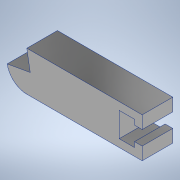
# Autodesk Inventor part: Finray_test_8
Saved by Autodesk Inventor 2022 (Build 260153000, 153)
## iProperties
Created: 2022-02-28
Part Number: Finray_test_8
Material: Generic
Document SubType Name: Modeling
Designer: richa
Density: 1 g/cm^3
Appearance: Aluminum - Flat
Author: richa
Autodesk Inventor part; units mm, degrees
ref_plane "YZ Plane" through (0, 0, 0) normal (1, 0, 0) x (0, 1, 0)
ref_plane "XZ Plane" through (0, 0, 0) normal (0, 1, 0) x (-1, 0, 0)
ref_plane "XY Plane" through (0, 0, 0) normal (0, 0, 1) x (1, 0, 0)
sketch "Sketch5" plane through (0, 0, 0) normal (0, 0, 1) x (1, 0, 0)
  line L0 (53, -15.6) -> (53, -10.6)
  line L1 (53, -10.6) -> (50, -10.6)
  line L2 (50, -10.6) -> (50, -12.6)
  line L3 (44, -12.6) -> (44, -3)
  line L4 (50, -3) -> (50, -5)
  line L5 (50, -5) -> (53, -5)
  line L6 (53, -5) -> (53, 0)
  line L7 (53, 0) -> (7.8, 0)
  line L8 (44, -3) -> (50, -3)
  line L9 (44, -12.6) -> (50, -12.6)
  line L10 (53, -15.6) -> (7.8, -15.6)
  arc A0 (7.8, 0) -> (7.8, -15.6) centre (7.8, -7.8) ccw
  point P0 (0, 0)
  dimension "d41" = 6
  dimension "d48" = 44
  dimension "d50" = 3
  dimension "d63" = 45.2
  dimension "d67" = 15.6
  dimension "d71" = 0
  dimension "d72" = 36.2
  dimension "d73" = 5
  dimension "d75" = 5
  dimension "d76" = 3
  dimension "d77" = 3
  constraints: 22 end point, 7 perpendicular, 2 collinear, 2 parallel, 2 point on circle, 2 tangent, 1 centre point, 1 horizontal, 1 vertical
  measures "d41" distance between parallel lines of L2 L3
  measures "d48" distance from line of L3 point (0, 0)
  measures "d50" distance of L4.end L5.end
  measures "d63" distance of L0.start L10.end
  measures "d67" diameter of A0
  measures "d71" distance from line of point (0, 0) L7
  measures "d72" distance from line of L3 A0.centre
  measures "d73" distance of L0.start L0.end
  measures "d75" distance of L5.end L6.end
  measures "d76" distance between parallel lines of L10 L9
  measures "d77" distance between parallel lines of L8 L7
extrude "Extrusion2" add sketch "Sketch5" along normal blind 12
sketch "Sketch8" plane through (0, 0, 0) normal (0, 0, -1) x (-1, 0, 0)
  arc A0 (-7.8, -15.6) -> (-7.8, 0) centre (-7.8, -7.8) ccw projected
  line L0 (-7.8, 0) -> (-9.1339, -7.5648)
  line L1 (-7.8, 0) -> (-1.143, 0) construction
  line L2 (-9.1339, -7.5648) -> (-0.1185, -9.1545)
  arc A1 (-7.8, -15.6) -> (-7.8, 0) centre (-7.8, -7.8) ccw projected
  line L3 (-7.8, -7.8) -> (4.6142, -7.8) construction
  line L4 (1.4517, -9.4313) -> (-7.8, -7.8) construction
  line L5 (-7.8, -7.8) -> (-18.1105, -5.982) construction
  line L6 (-53, 0) -> (-7.8, 0) projected
  arc A2 (-0.1185, -9.1545) -> (-7.8, 0) centre (-7.8, -7.8) ccw
  point P0 (0, 0)
  point P1 (-0.1185, -9.1545)
  dimension "d80" = 100
  dimension "d81" = 10
  constraints: 12 end point, 3 point on circle, 2 horizontal, 2 point on line, 1 centre point, 1 concentric, 1 perpendicular
  measures "d80" angle of L0 L1
  measures "d81" angle of L3 L4
extrude "Extrusion5" cut sketch "Sketch8" against normal through all
equation "\"l1\" = 8"
body "Solid2"
